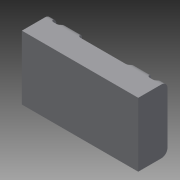
# Autodesk Inventor part: holder
Saved by Autodesk Inventor 2014 (Build 180170000, 170)
## iProperties
Created: 2013-06-25
Part Number: holder
Material: Generisch
Document SubType Name: Modeling
Designer: Felix
Density: 1 g/cm^3
Appearance: Vorgabe
Author: Felix
Autodesk Inventor part; units mm, degrees
ref_plane "YZ Plane" through (0, 0, 0) normal (1, 0, 0) x (0, 1, 0)
ref_plane "XZ Plane" through (0, 0, 0) normal (0, 1, 0) x (-1, 0, 0)
sketch "Skizze1" plane through (0, 0, 0) normal (0, 1, 0) x (-1, 0, 0)
  line L0 (0, 0) -> (75.5, 0)
  line L1 (75.5, 0) -> (75.5, 41.5)
  line L2 (75.5, 41.5) -> (0, 41.5)
  line L3 (0, 41.5) -> (0, 0)
  dimension "d0" = 75.5
  dimension "d1" = 41.5
  constraints: 8 end point, 2 parallel, 1 horizontal, 1 perpendicular
  measures "d0" distance of L2.end L1.end
  measures "d1" distance of L1.end L0.end
extrude "Extrusion1" add sketch "Skizze1" along normal blind 19
ref_plane "Arbeitsebene1" through (-37.75, 0, 41.5) normal (1, 0, 0) x (0, 0, -1)
fillet "Rundung2" radius 4 2 edges at (-37.75, 19, 41.5) (-37.75, 19, 0)
shell "Hülle1" thickness 2 removed faces 0
sketch "Skizze2" plane through (-75.5, 0, 41.5) normal (0, 0, 1) x (1, 0, 0)
  line L0 (0, 0) -> (75.5, 0) projected
  line L1 (75.5, 0) -> (75.5, 19) projected
  line L2 (0, 19) -> (75.5, 19) projected
  line L3 (0, 0) -> (0, 19) projected
  line L4 (5.4864, 15) -> (7.5307, 15)
  line L5 (3.4864, 19) -> (3.4864, 17)
  line L6 (20.9731, 17) -> (20.9731, 17)
  line L7 (0, 19) -> (3.4864, 19)
  line L8 (9.5307, 17) -> (9.5307, 17)
  arc A0 (3.4864, 17) -> (5.4864, 15) centre (5.4864, 17) ccw
  arc A1 (7.5307, 15) -> (9.5307, 17) centre (7.5307, 17) ccw
  line L9 (11.5307, 19) -> (18.9731, 19)
  arc A2 (11.5307, 19) -> (9.5307, 17) centre (11.5307, 17) ccw
  arc A3 (20.9731, 17) -> (18.9731, 19) centre (18.9731, 17) ccw
  line L10 (22.9731, 15) -> (37.75, 15)
  line L11 (37.75, 19) -> (18.9731, 19)
  line L12 (37.75, 15) -> (37.75, 19)
  arc A4 (20.9731, 17) -> (22.9731, 15) centre (22.9731, 17) ccw
  point P0 (0, 15)
  point P1 (75.5, 15)
  point P2 (20.9731, 19)
  point P3 (20.9731, 15)
  point P4 (9.5307, 19)
  dimension "d4" = 4
  dimension "d5" = 2
  dimension "d6" = 2
  dimension "d7" = 2
  dimension "d8" = 2
  constraints: 18 end point, 14 point on line, 11 tangent, 10 point on circle, 5 centre point, 5 perpendicular, 3 collinear, 1 equal radius, 1 midpoint, 1 parallel
  measures "d4" distance between parallel lines of L2 L4
  measures "d5" radius of A0
  measures "d6" radius of A1
  measures "d7" radius of A2
  measures "d8" radius of A4
extrude "Extrusion2" cut sketch "Skizze2" against normal through all contours L2 A2 A1 L4 A0 L5 | L12 L10 A4 A3 L2
mirror "Spiegeln1" about plane through (-37.75, 0, 41.5) normal (1, 0, 0) of "Extrusion2"
sketch "Skizze3" plane through (0, 19, 0) normal (0, 1, 0) x (1, 0, 0)
  line L0 (-75.5, -4) -> (-75.5, -37.5) projected
  line L1 (0, -37.5) -> (0, -4) projected
  line L2 (0, 0) -> (-75.5, 0) projected
  line L3 (-75.5, -41.5) -> (0, -41.5) projected
  line L4 (-75.5, 0) -> (-75.5, -41.5) projected
  line L5 (0, -41.5) -> (0, 0) projected
  line L6 (-73.5, -4) -> (-2, -4)
  line L7 (-2, -4) -> (-2, -37.5)
  line L8 (-2, -37.5) -> (-73.5, -37.5)
  line L9 (-73.5, -37.5) -> (-73.5, -4)
  point P0 (-58, -2)
  point P1 (-58, -39.5)
  point P2 (0, -39.5)
  point P3 (0, -2)
  point P4 (-58, -0.0331)
  point P5 (-58, -41.4669)
  point P6 (0, -41.4669)
  point P7 (0, -0.0331)
  point P8 (-75.5, -37.5)
  dimension "d13" = 2
  dimension "d14" = 2
  dimension "d15" = 4
  dimension "d16" = 4
  constraints: 8 end point, 2 parallel, 1 horizontal, 1 perpendicular, 2 other
  measures "d13" distance between parallel lines of L1 L7
  measures "d15" distance between parallel lines of L2 L6
  measures "d16" distance between parallel lines of L3 L8
extrude "Extrusion3" cut sketch "Skizze3" against normal up to surface (17 mm away) contours L6 L7 L8 L9
sketch "Skizze4" plane through (-73.5, 2, 2) normal (0, 1, 0) x (1, 0, 0)
  line L0 (71.5, -37.5) -> (71.5, 0) projected
  line L1 (71.5, 0) -> (0, 0) projected
  line L2 (0, 0) -> (0, -37.5) projected
  line L3 (0, -37.5) -> (71.5, -37.5) projected
  line L4 (0, -18) -> (71.5, -18)
  line L5 (71.5, -18) -> (71.5, -19.5)
  line L6 (71.5, -19.5) -> (0, -19.5)
  line L7 (0, -19.5) -> (0, -18)
  line L8 (35.75, -18) -> (35.75, 0)
  line L9 (35.75, -19.5) -> (35.75, -37.5)
  point P0 (73.5, 2)
  dimension "d20" = 1.5
  constraints: 12 end point, 4 midpoint, 2 parallel, 2 point on line, 1 collinear, 1 horizontal, 1 perpendicular
  measures "d20" distance between parallel lines of L4 L6
extrude "Extrusion4" add sketch "Skizze4" along normal up to surface (13 mm away) contours L6 L2 L4 L0
sketch "Skizze5" plane through (-73.5, 2, 2) normal (1, 0, 0) x (0, 0, -1)
  line L0 (-19.5, 0) -> (-19.5, 13) projected
  line L1 (-19.5, 13) -> (-18, 13) projected
  line L2 (-18, 13) -> (-18, 0) projected
  line L3 (0, 0) -> (-18, 0) projected
  line L4 (0, 0) -> (0, 13) projected
  arc A0 (0, 13) -> (-2, 15) centre (-2, 13) ccw projected
  line L5 (-2, 17) -> (-2, 15) projected
  line L6 (-35.5, 17) -> (-2, 17) projected
  line L7 (-35.5, 17) -> (-35.5, 15) projected
  arc A1 (-35.5, 15) -> (-37.5, 13) centre (-35.5, 13) ccw projected
  line L8 (-37.5, 0) -> (-37.5, 13) projected
  line L9 (-19.5, 0) -> (-37.5, 0) projected
  circle A2 centre (-28.5, 9) radius 9
  circle A3 centre (-9, 9) radius 9
  point P0 (2, -2)
  constraints: 6 tangent, 2 centre point
